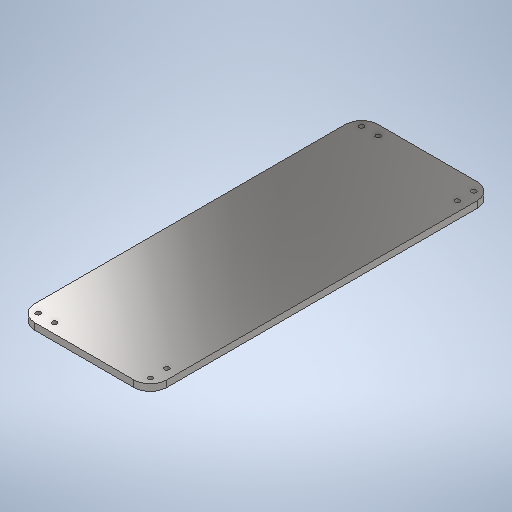
# Autodesk Inventor part: Mid_plate
Saved by Autodesk Inventor 2025.2 (Build 292293000, 293)
## iProperties
Created: 2025-02-20
Part Number: Mid_plate
Material: Stainless Steel
Document SubType Name: Modeling
Designer: Sergio Quintero
Density: 8 g/cm^3
Appearance: Semi-Polished
Mass: 8245.1 g
Surface Area: 2223.4 cm^2
Volume: 1030.64 cm^3
Author: Sergio Quintero
Autodesk Inventor part; units mm, degrees
note: some values were not read from the file. Chosen so that the rebuilt part matches the saved one: pattern direction of "Rectangular Pattern1".
ref_plane "YZ Plane" through (0, 0, 0) normal (1, 0, 0) x (0, 1, 0)
ref_plane "XZ Plane" through (0, 0, 0) normal (0, 1, 0) x (-1, 0, 0)
ref_plane "XY Plane" through (0, 0, 0) normal (0, 0, 1) x (1, 0, 0)
sketch "Sketch1" plane through (0, 0, 0) normal (0, 1, 0) x (-1, 0, 0)
  line L0 (-100, -260) -> (100, -260)
  line L1 (100, -260) -> (100, 260)
  line L2 (100, 260) -> (-100, 260)
  line L3 (-100, 260) -> (-100, -260)
  line L4 (-100, -260) -> (100, 260) construction
  line L5 (100, -260) -> (-100, 260) construction
  point P0 (0, 0)
  dimension "d0" = 200
  dimension "d1" = 520
  constraints: 12 end point, 2 midpoint, 2 parallel, 1 horizontal, 1 perpendicular
  measures "d0" distance of L2.end L1.end
  measures "d1" distance of L1.end L0.end
extrude "Extrusion1" add sketch "Sketch1" along normal blind 10
fillet "Fillet1" radius 25 4 edges at (-100, 5, -260) (-100, 5, 260) (100, 5, 260) (100, 5, -260)
sketch "Sketch2" plane through (0, 10, 0) normal (0, 1, 0) x (1, 0, 0)
  line L0 (100, -235) -> (100, 235) projected
  line L1 (-75, -260) -> (75, -260) projected
  point P0 (0, 0)
  point P1 (85, -245)
  dimension "d5" = 15
  dimension "d6" = 15
  measures "d5" distance from line of L0 point (85, -245)
  measures "d6" distance from line of point (85, -245) L1
hole "Hole1" at (85, 10, 245) direction (0, -1, 0) diameter 7.134 end through all thread size "M8x0.8" class "6H" standard "ISO Metric profile"
pattern_linear "Rectangular Pattern1" count 2 spacing 170 along (-1, 0, 0) count 2 spacing 490 along (0, 0, -1) of "Hole1"
sketch "Sketch7" plane through (0, 10, 0) normal (0, 1, 0) x (1, 0, 0)
  circle A0 centre (85, -245) radius 3.567 projected
  line L0 (100, -235) -> (100, 235) projected
  circle A1 centre (-85, -245) radius 3.567 projected
  line L1 (-75, -260) -> (75, -260) projected
  point P0 (0, 0)
  point P1 (85, -220)
  point P2 (-60, -245)
  dimension "d61" = 25
  dimension "d62" = 15
  dimension "d63" = 25
  dimension "d64" = 15
  measures "d61" distance of A0.centre point (85, -220)
  measures "d62" distance from line of L0 point (85, -220)
  measures "d63" distance of A1.centre point (-60, -245)
  measures "d64" distance from line of point (-60, -245) L1
hole "Hole6" at (85, 10, 220) at (-60, 10, 245) direction (0, -1, 0) diameter 7.134 end through all thread size "M8x0.8" class "6H" standard "ISO Metric profile"
mirror "Mirror2" about plane through (0, 0, 0) normal (0, 0, 1) of "Hole6"
body "Solid1"
